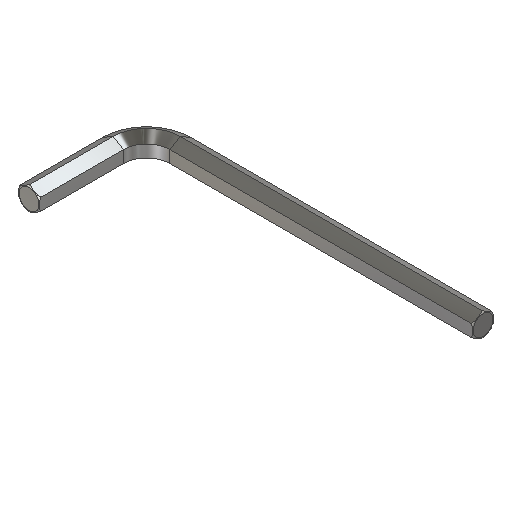
# Autodesk Inventor part: Allen 5 mm
Saved by Autodesk Inventor 2025.2 (Build 292293000, 293)
## iProperties
Created: 2018-02-09
Part Number: Allen 5 mm
Material: Acero inoxidable AISI 304
Document SubType Name: Modeling
Designer: T.S.U Miguel González
Mass: 18.0941 g
Surface Area: 18.5188 cm^2
Volume: 2.26176 cm^3
Density: 8 g/cm^3
Appearance: Cromo - Pulido
Author: T.S.U Miguel González
Autodesk Inventor part; units mm, degrees
ref_plane "YZ Plane" through (0, 0, 0) normal (1, 0, 0) x (0, 1, 0)
ref_plane "XZ Plane" through (0, 0, 0) normal (0, 1, 0) x (-1, 0, 0)
sketch "Boceto1" plane through (0, 0, 0) normal (0, 1, 0) x (-1, 0, 0)
  circle A0 centre (0, 0) radius 2.495 construction
  circle A1 centre (0, 0) radius 2 construction
  line L0 (2.495, -1.4405) -> (0, -2.881)
  line L1 (0, -2.881) -> (-2.495, -1.4405)
  line L2 (-2.495, -1.4405) -> (-2.495, 1.4405)
  line L3 (-2.495, 1.4405) -> (0, 2.881)
  line L4 (0, 2.881) -> (2.495, 1.4405)
  line L5 (2.495, 1.4405) -> (2.495, -1.4405)
  point P0 (2.495, 0)
  dimension "d0" = 4.99
  dimension "d1" = 4
  constraints: 12 end point, 3 coincident, 1 centre point, 1 horizontal alignment, 1 midpoint, 15 other
  measures "d1" diameter of A1
sketch "Boceto2" plane through (0, 0, 0) normal (0, 0, 1) x (1, 0, 0)
  line L0 (0, 0) -> (0, 20)
  line L1 (8, 28) -> (80, 28)
  arc A0 (8, 28) -> (0, 20) centre (8, 20) ccw
  constraints: 4 end point, 2 point on circle, 1 centre point, 1 perpendicular, 1 vertical
sweep "Barrido1" add profiles "Boceto1" path "Boceto2"
sketch "Boceto3" plane through (0, 0, 0) normal (1, 0, 0) x (0, 1, 0)
  line L0 (26.793, 1.4405) -> (26.793, -1.4405) projected
  line L1 (20, -2.881) -> (0, -2.881) projected
  line L2 (0, -2.881) -> (0, 2.881) projected
  line L3 (0, 2.881) -> (20, 2.881) projected
  arc A0 (0.5, 2.881) -> (0, 2.381) centre (0.5, 2.381) ccw
  line L4 (0, 2.381) -> (-0.2924, 2.381)
  line L5 (-0.2924, 2.381) -> (-0.2924, 3.2696)
  line L6 (-0.2924, 3.2696) -> (0.5, 3.2696)
  line L7 (0.5, 3.2696) -> (0.5, 2.881)
  line L8 (0, 0) -> (-2.0154, 0)
  constraints: 10 end point, 3 perpendicular, 2 horizontal, 2 point on circle, 1 centre point, 2 other
revolve "Revolución1" cut sketch "Boceto3" angle 360 about axis through (0, 0, 0) along (0, -1, 0)
ref_plane "Plano de trabajo1" through (8, 28, 2.881) normal (0, 1, 0) x (1, 0, 0)
sketch "Boceto4" plane through (8, 28, 2.881) normal (0, 1, 0) x (1, 0, 0)
  line L0 (72, 0) -> (0, 0) construction
  line L1 (-6.793, 1.4405) -> (-6.793, 4.3215) construction
  line L2 (0, 5.762) -> (72, 5.762) construction
  line L3 (72, 5.762) -> (72, 0) construction
  line L4 (72, 1.4405) -> (72, 4.3215) projected
  line L5 (72, 2.881) -> (73.7446, 2.881)
  arc A0 (72, 5.262) -> (71.5, 5.762) centre (71.5, 5.262) ccw
  line L6 (72, 5.262) -> (72.3922, 5.262)
  line L7 (72.3922, 5.262) -> (72.3922, 6.043)
  line L8 (72.3922, 6.043) -> (71.5, 6.043)
  line L9 (71.5, 6.043) -> (71.5, 5.762)
  point P0 (-8, 2.881)
  constraints: 10 end point, 2 horizontal, 2 parallel, 2 point on circle, 1 centre point, 1 midpoint, 1 perpendicular, 2 other
revolve "Revolución2" cut sketch "Boceto4" angle 360 about axis through (80, 28, 0) along (1, 0, 0)
